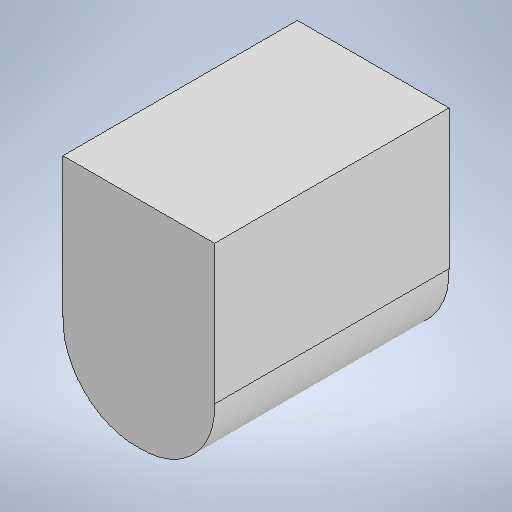
# Autodesk Inventor part: Horn
Saved by Autodesk Inventor 2025 (Build 290162000, 162)
## iProperties
Created: 2024-05-25
Part Number: Horn
Material: Generic
Document SubType Name: Modeling
Designer: hifzh
Density: 1 g/cm^3
Appearance: Default
Author: hifzh
Autodesk Inventor part; units mm, degrees
ref_plane "YZ Plane" through (0, 0, 0) normal (1, 0, 0) x (0, 1, 0)
ref_plane "XZ Plane" through (0, 0, 0) normal (0, 1, 0) x (-1, 0, 0)
ref_plane "XY Plane" through (0, 0, 0) normal (0, 0, 1) x (1, 0, 0)
sketch "Sketch1" plane through (0, 0, 0) normal (0, 0, 1) x (1, 0, 0)
  circle A0 centre (0, 0) radius 17.705
  circle A1 centre (0, 0) radius 15
  circle A2 centre (0, 15) radius 0.75
  circle A3 centre (-10.6066, 10.6066) radius 0.75
  circle A4 centre (0, 0) radius 15
  circle A5 centre (-15, 0) radius 0.75
  circle A6 centre (0, 0) radius 15
  circle A7 centre (-10.6066, -10.6066) radius 0.75
  circle A8 centre (0, 0) radius 15
  circle A9 centre (0, -15) radius 0.75
  circle A10 centre (0, 0) radius 15
  circle A11 centre (10.6066, -10.6066) radius 0.75
  circle A12 centre (0, 0) radius 15
  circle A13 centre (15, 0) radius 0.75
  circle A14 centre (0, 0) radius 15
  circle A15 centre (10.6066, 10.6066) radius 0.75
  circle A16 centre (0, 0) radius 15
  line L0 (-20.705, 38) -> (20.705, 38)
  arc A17 (0, -20.705) -> (20.705, 0) centre (0.7179, -0.7179) ccw
  arc A18 (-20.705, 0) -> (0, -20.705) centre (-0.7179, -0.7179) ccw
  line L1 (-20.705, 0) -> (-20.705, 38)
  line L2 (20.705, 38) -> (20.705, 0)
  dimension "d1" = 30
  dimension "d0" = 35.41
  dimension "d2" = 1.5
  dimension "d5" = 360
  dimension "d10" = 38
  dimension "d11" = 20
  dimension "d12" = 20
  dimension "d15" = 58.705
  constraints: 11 centre point, 6 end point, 4 coincident, 4 point on circle, 2 horizontal alignment, 2 vertical alignment, 1 horizontal, 1 parallel, 1 vertical, 51 other
  measures "d0" diameter of A0
  measures "d2" diameter of A2
  measures "d10" distance from line of A0.centre L0
  measures "d11" radius of A17
  measures "d12" radius of A18
  measures "d15" distance from line of A17.start L0
sketch "Sketch2" plane through (0, 0, 0) normal (0, 0, 1) x (1, 0, 0)
  point P0 (0, 0)
sketch "Sketch3" plane through (0, 0, 0) normal (0, 0, 1) x (1, 0, 0)
  point P0 (0, 0)
sketch "Sketch4" plane through (0, 0, 0) normal (0, 0, 1) x (1, 0, 0)
  point P0 (0, 0)
extrude "Extrusion1" add sketch "Sketch1" along normal mid plane 64 contours A0 | A1 A13 | A1 A13 | A13 A1 A11 A9 A7 A5 A3 A2 A15 | A15 A1 | A1 A15 | A11 A1 | A1 A11 | A2 A1 | A1 A2 | A9 A1 | A1 A9 | A3 A1 | A1 A3 | A7 A1 | A1 A7 | A5 A1 | A1 A5 | L0 L2 A17 A18 L1
body "Solid1"
